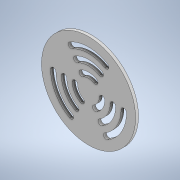
# Autodesk Inventor part: Моя пластина
Saved by Autodesk Inventor 2021 (Build 250183000, 183)
## iProperties
Created: 2020-11-09
Part Number: Моя пластина
Material: Типовые
Document SubType Name: Modeling
Designer: Тимоха
Density: 1 g/cm^3
Appearance: По умолчанию
Author: Тимоха
Autodesk Inventor part; units mm, degrees
ref_plane "YZ Plane" through (0, 0, 0) normal (1, 0, 0) x (0, 1, 0)
ref_plane "XZ Plane" through (0, 0, 0) normal (0, 1, 0) x (-1, 0, 0)
ref_plane "XY Plane" through (0, 0, 0) normal (0, 0, 1) x (1, 0, 0)
sketch "Эскиз1" plane through (0, 0, 0) normal (0, 0, 1) x (1, 0, 0)
  circle A0 centre (0, 0) radius 65
  dimension "d0" = 130
  constraints: 1 centre point, 1 coincident
  measures "d0" diameter of A0
extrude "Выдавливание1" add sketch "Эскиз1" along normal blind 4
sketch "Эскиз2" plane through (0, 0, 4) normal (0, 0, 1) x (1, 0, 0)
  line L0 (-91, 0) -> (91, 0) projected
  line L1 (0, -91) -> (0, 91) projected
  arc A0 (7.5, 12.9904) -> (11.25, 19.4856) centre (9.375, 16.238) ccw
  arc A1 (15, 25.9808) -> (18.75, 32.476) centre (16.875, 29.2284) ccw
  arc A2 (22.5, 38.9711) -> (26.25, 45.4663) centre (24.375, 42.2187) ccw
  arc A3 (-11.25, 19.4856) -> (-7.5, 12.9904) centre (-9.375, 16.238) ccw
  arc A4 (-18.75, 32.476) -> (-15, 25.9808) centre (-16.875, 29.2284) ccw
  arc A5 (-26.25, 45.4663) -> (-22.5, 38.9711) centre (-24.375, 42.2187) ccw
  arc A6 (7.5, 12.9904) -> (-7.5, 12.9904) centre (0, 0) ccw
  arc A7 (11.25, 19.4856) -> (-11.25, 19.4856) centre (0, 0) ccw
  arc A8 (15, 25.9808) -> (-15, 25.9808) centre (0, 0) ccw
  arc A9 (18.75, 32.476) -> (-18.75, 32.476) centre (0, 0) ccw
  arc A10 (22.5, 38.9711) -> (-22.5, 38.9711) centre (0, 0) ccw
  arc A11 (26.25, 45.4663) -> (-26.25, 45.4663) centre (0, 0) ccw
  arc A12 (-52.5, 0) -> (-26.25, -45.4663) centre (0, 0) ccw
  arc A13 (-45, 0) -> (-22.5, -38.9711) centre (0, 0) ccw
  arc A14 (-26.25, -45.4663) -> (-22.5, -38.9711) centre (-24.375, -42.2187) ccw
  arc A15 (-45, 0) -> (-52.5, 0) centre (-48.75, 0) ccw
  arc A16 (-30, 0) -> (-37.5, 0) centre (-33.75, 0) ccw
  arc A17 (-37.5, 0) -> (-18.75, -32.476) centre (0, 0) ccw
  arc A18 (-30, 0) -> (-15, -25.9808) centre (0, 0) ccw
  arc A19 (-18.75, -32.476) -> (-15, -25.9808) centre (-16.875, -29.2284) ccw
  arc A20 (-22.5, 0) -> (-11.25, -19.4856) centre (0, 0) ccw
  arc A21 (-15, 0) -> (-7.5, -12.9904) centre (0, 0) ccw
  arc A22 (-11.25, -19.4856) -> (-7.5, -12.9904) centre (-9.375, -16.238) ccw
  arc A23 (-15, 0) -> (-22.5, 0) centre (-18.75, 0) ccw
  arc A24 (26.25, -45.4663) -> (52.5, 0) centre (0, 0) ccw
  arc A25 (22.5, -38.9711) -> (45, 0) centre (0, 0) ccw
  arc A26 (52.5, 0) -> (45, 0) centre (48.75, 0) ccw
  arc A27 (22.5, -38.9711) -> (26.25, -45.4663) centre (24.375, -42.2187) ccw
  arc A28 (15, -25.9808) -> (18.75, -32.476) centre (16.875, -29.2284) ccw
  arc A29 (18.75, -32.476) -> (37.5, 0) centre (0, 0) ccw
  arc A30 (15, -25.9808) -> (30, 0) centre (0, 0) ccw
  arc A31 (37.5, 0) -> (30, 0) centre (33.75, 0) ccw
  arc A32 (11.25, -19.4856) -> (22.5, 0) centre (0, 0) ccw
  arc A33 (7.5, -12.9904) -> (15, 0) centre (0, 0) ccw
  arc A34 (22.5, 0) -> (15, 0) centre (18.75, 0) ccw
  arc A35 (7.5, -12.9904) -> (11.25, -19.4856) centre (9.375, -16.238) ccw
  circle A36 centre (0, 0) radius 14
  dimension "d12" = 360
  dimension "d24" = 28
  constraints: 72 point on circle, 37 centre point, 17 coincident, 9 symmetric about line, 112 other
  measures "d24" diameter of A36
extrude "Выдавливание2" cut sketch "Эскиз2" against normal through all contours A15 L0 | L0 A13 A14 A12 | A10 A5 A11 L1 | L1 A11 A2 A10 | A8 A4 A9 L1 | L1 A9 A1 A8 | A6 A3 A7 L1 | L1 A7 A0 A6 | A26 L0 | L0 A24 A27 A25 | A31 L0 | L0 A29 A28 A30 | A34 L0 | L0 A32 A35 A33 | A23 L0 | L0 A21 A22 A20 | A16 L0 | L0 A18 A19 A17
